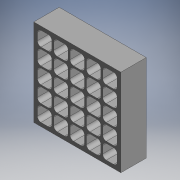
# Autodesk Inventor part: Cavity Lattice Demo
Saved by Autodesk Inventor 2019 (Build 230136000, 136)
## iProperties
Part Number: Cavity Lattice Demo
Material: Generic
Document SubType Name: Modeling
Designer: oriani
Appearance: Default
Author: oriani
Autodesk Inventor part; units mm, degrees
ref_plane "YZ Plane" through (0, 0, 0) normal (1, 0, 0) x (0, 1, 0)
ref_plane "XZ Plane" through (0, 0, 0) normal (0, 1, 0) x (-1, 0, 0)
ref_plane "XY Plane" through (0, 0, 0) normal (0, 0, 1) x (1, 0, 0)
sketch "Sketch1" plane through (0, 0, 0) normal (0, 0, 1) x (1, 0, 0)
  line L0 (0, 0) -> (-152.4, 0)
  line L1 (-152.4, 0) -> (-152.4, 152.4)
  line L2 (-152.4, 152.4) -> (0, 152.4)
  line L3 (0, 152.4) -> (0, 0)
  line L4 (-36.5125, 19.05) -> (-30.1625, 19.05) construction
  line L5 (-36.5125, 17.4625) -> (-30.1625, 17.4625)
  line L6 (-30.1625, 20.6375) -> (-36.5125, 20.6375)
  arc A0 (-36.5125, 20.6375) -> (-36.5125, 17.4625) centre (-36.5125, 19.05) ccw
  arc A1 (-30.1625, 17.4625) -> (-30.1625, 20.6375) centre (-30.1625, 19.05) ccw
  line L7 (-19.05, 30.1625) -> (-19.05, 36.5125) construction
  line L8 (-17.4625, 30.1625) -> (-17.4625, 36.5125)
  line L9 (-20.6375, 36.5125) -> (-20.6375, 30.1625)
  arc A2 (-20.6375, 30.1625) -> (-17.4625, 30.1625) centre (-19.05, 30.1625) ccw
  arc A3 (-17.4625, 36.5125) -> (-20.6375, 36.5125) centre (-19.05, 36.5125) ccw
  point P0 (-33.3375, 19.05)
  point P1 (-19.05, 33.3375)
  constraints: 24 end point, 8 point on circle, 8 tangent, 4 centre point, 2 midpoint, 2 parallel
sketch "Sketch2" plane through (0, 0, 6.35) normal (0, 0, 1) x (1, 0, 0)
  line L0 (-6.35, 12.7) -> (-6.35, 25.4)
  arc A0 (-6.35, 25.4) -> (-12.7, 31.75) centre (-12.7, 25.4) ccw
  line L1 (-12.7, 31.75) -> (-25.4, 31.75)
  arc A1 (-25.4, 31.75) -> (-31.75, 25.4) centre (-25.4, 25.4) ccw
  line L2 (-31.75, 25.4) -> (-31.75, 12.7)
  arc A2 (-31.75, 12.7) -> (-25.4, 6.35) centre (-25.4, 12.7) ccw
  line L3 (-25.4, 6.35) -> (-12.7, 6.35)
  arc A3 (-12.7, 6.35) -> (-6.35, 12.7) centre (-12.7, 12.7) ccw
  circle A4 centre (-19.05, 22.7162) radius 1.5875
  circle A5 centre (-22.225, 17.2169) radius 1.5875
  circle A6 centre (-15.875, 17.2169) radius 1.5875
  constraints: 8 end point, 8 point on circle, 7 centre point
extrude "Extrusion1" add sketch "Sketch1" along normal blind 44.45 contours L0 L1 L2 L3 | A0 L6 A1 L5 | A2 L9 A3 L8
extrude "Extrusion2" cut sketch "Sketch1" along normal blind 9.525 contours A0 L6 A1 L5
extrude "Extrusion3" cut sketch "Sketch1" along normal blind 9.525 contours A2 L9 A3 L8
extrude "Extrusion4" cut sketch "Sketch2" along normal blind 38.1 contours A3 L3 A2 L2 A1 L1 A0 L0 | A4 | A5 | A6
extrude "Extrusion5" add sketch "Sketch2" along normal blind 6.35 contours A4
extrude "Extrusion6" add sketch "Sketch2" along normal blind 6.35 contours A5
extrude "Extrusion7" add sketch "Sketch2" along normal blind 6.35 contours A6
pattern_linear "Rectangular Pattern1" count 5 spacing 28.575 along (-1, 0, 0) of "Extrusion4", "Extrusion5", "Extrusion6", "Extrusion7"
pattern_linear "Rectangular Pattern2" count 5 spacing 28.575 along (0, 1, 0) of "Extrusion4", "Extrusion5", "Extrusion6", "Extrusion7", "Rectangular Pattern1"
pattern_linear "Rectangular Pattern3" count 4 spacing 28.575 along (-1, 0, 0) of "Extrusion2"
pattern_linear "Rectangular Pattern4" count 5 spacing 28.575 along (0, 1, 0) of "Extrusion2", "Rectangular Pattern3"
pattern_linear "Rectangular Pattern5" count 5 spacing 28.575 along (-1, 0, 0) of "Extrusion3"
pattern_linear "Rectangular Pattern6" count 4 spacing 28.575 along (0, 1, 0) of "Extrusion3", "Rectangular Pattern5"
body "Solid1"
